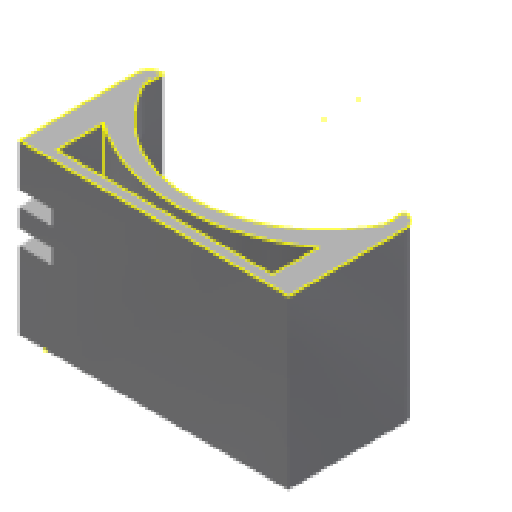
# Autodesk Inventor part: Gehäuse_Kurve
Saved by Autodesk Inventor 2023 (Build 270158000, 158)
## iProperties
Created: 2025-01-24
Part Number: Gehäuse_Kurve
Material: ABS-Kunststoff
Document SubType Name: Modeling
Designer: abdel
Density: 1.06 g/cm^3
Appearance: Glatt - Weiß
Author: abdel
Autodesk Inventor part; units mm, degrees
ref_plane "YZ Plane" through (0, 0, 0) normal (1, 0, 0) x (0, 1, 0)
ref_plane "XY Plane" through (0, 0, 0) normal (0, 0, 1) x (1, 0, 0)
sketch "Skizze1" plane through (0, 0, 0) normal (0, 0, 1) x (1, 0, 0)
  line L0 (20, 16.3) -> (20, 0)
  line L1 (20, 0) -> (-20, 0)
  line L2 (-20, 0) -> (-20, 16.3)
  line L3 (-16, 8.4971) -> (-16, 1.5701)
  line L4 (-16, 1.5701) -> (16, 1.5701)
  line L5 (16, 1.5701) -> (16, 8.4971)
  line L6 (-20, 16.3) -> (-17.85, 16.3)
  line L7 (20, 16.3) -> (17.85, 16.3)
  arc A0 (-16, 8.4971) -> (16, 8.4971) centre (0, 30.4255) ccw
  arc A1 (-17.85, 16.3) -> (17.85, 16.3) centre (0, 25.395) ccw
  line L8 (2.1309, 0) -> (0, 0)
  line L9 (0, 16.2928) -> (2.1309, 16.2928)
  line L10 (2.1309, 16.2928) -> (2.1309, 0)
  line L11 (2.1309, 0) -> (0, 0)
  line L12 (0, 0) -> (0, 16.2928)
  line L13 (37.8691, 16.2928) -> (40, 16.2928)
  line L14 (40, 16.2928) -> (40, 0)
  line L15 (40, 0) -> (37.8691, 0)
  line L16 (37.8691, 0) -> (37.8691, 16.2928)
  line L17 (0, 0) -> (40, 0)
  line L18 (0, 0) -> (0, 12.8953)
  line L19 (40, 0) -> (40, 79)
  arc A2 (2.1309, 16.2928) -> (37.8691, 16.2928) centre (20, 25.8644) ccw
  line L20 (6.1071, 11.1028) -> (5.3563, 11.7632)
  point P0 (0, 8.1464)
  dimension "d27" = 40
  dimension "d28" = 4
  dimension "d58" = 16.3
  dimension "d60" = 126
  dimension "d61" = 2.15
  dimension "d62" = 2.1309
  constraints: 42 end point, 7 point on circle, 6 horizontal, 5 parallel, 4 equal length, 4 point on line, 3 centre point, 3 vertical, 2 midpoint, 2 perpendicular, 1 coincident
  measures "d27" distance of L0.end L1.end
  measures "d28" distance between parallel lines of L0 L5
  measures "d58" distance of L1.end L2.end
  measures "d61" distance of L2.end L6.end
  measures "d62" distance of L9.start L9.end
extrude "Extrusion1" add sketch "Skizze1" along normal blind 25 contours L0 A2 L5 A0 A1 L7 | L0 L1 L10 L4 L5 A2 | A2 A0 L10 A1 | L1 L12 L4 L10 | L10 A0 L12 A1 | L1 L2 L6 A1 L12 A0 L3 L4
sketch "Skizze2" plane through (-20, 16.3, 0) normal (0, 1, 0) x (1, 0, 0)
  line L0 (2.15, 0) -> (0, 0) projected
  line L1 (0, 0) -> (0, -25) projected
  line L2 (2.15, -25) -> (0, -25) projected
  line L3 (2.15, 0) -> (2.15, -25) projected
  point P0 (20, 0)
extrude "Extrusion2" add sketch "Skizze2" along normal blind 3
sketch "Skizze3" plane through (17.85, 16.3, 0) normal (0, 1, 0) x (1, 0, 0)
  line L0 (2.15, 0) -> (0, 0) projected
  line L1 (0, 0) -> (0, -25) projected
  line L2 (2.15, -25) -> (0, -25) projected
  line L3 (2.15, 0) -> (2.15, -25) projected
  point P0 (-17.85, 0)
ref_plane "Arbeitsebene2" through (0, 10, 0) normal (0, 1, 0) x (-1, 0, 0)
extrude "Extrusion3" add sketch "Skizze3" along normal blind 3
sketch "Skizze4" plane through (0, 10, 0) normal (0, 1, 0) x (-1, 0, 0)
  line L0 (-17.85, 0) -> (-17.85, 25) projected
  line L1 (-17.85, 0) -> (17.85, 0) projected
  line L2 (17.85, 0) -> (17.85, 25) projected
  line L3 (-17.85, 25) -> (17.85, 25) projected
  line L4 (-17.85, 0) -> (-17.85, 25) projected
  line L5 (-17.85, 11.4) -> (17.85, 11.4)
  line L6 (-17.85, 13.65) -> (17.85, 13.65)
  line L7 (-17.85, 16.4) -> (17.85, 16.4)
  line L8 (-17.85, 18.65) -> (17.85, 18.65)
  line L9 (-17.85, 25) -> (-20, 25) projected
  point P0 (0, 0)
  point P1 (-17.85, 13.65)
  point P2 (-17.85, 11.4)
  point P3 (-17.85, 18.65)
  point P4 (-17.85, 16.4)
  dimension "d13" = 2.25
  dimension "d14" = 2.25
  dimension "d15" = 25
  dimension "d16" = 2.75
  dimension "d36" = 6.35
  constraints: 8 end point, 8 point on line, 4 horizontal
  measures "d13" distance between parallel lines of L5 L6
  measures "d14" distance between parallel lines of L7 L8
  measures "d15" distance between parallel lines of L1 L3
  measures "d16" distance between parallel lines of L6 L7
  measures "d36" distance between parallel lines of L9 L8
extrude "Extrusion4" cut sketch "Skizze4" along normal mid plane 14 contours L0 L6 L2 L5 | L0 L8 L2 L7
fillet "Rundung2" radius 2 2 edges at (-20, 19.3, 12.5) (20, 19.3, 12.5)
sketch "Skizze5" plane through (-16, 1.5701, 0) normal (1, 0, 0) x (0, 0, -1)
  line L0 (0, 0) -> (0, 6.927) projected
  line L1 (0, 6.927) -> (-25, 6.927) projected
  line L2 (-25, 0) -> (-25, 6.927) projected
  line L3 (0, 0) -> (-25, 0) projected
  point P0 (0, -1.5701)
sketch "Skizze12" plane through (-20, 0, 0) normal (-1, 0, 0) x (0, 0, 1)
  line L0 (0, 0) -> (25, 0) projected
  line L1 (18.65, 6.5) -> (18.65, 12)
  line L2 (13.65, 6.5) -> (13.65, 12)
  line L3 (18.65, 12) -> (16.4, 12)
  line L4 (16.4, 12) -> (16.4, 0)
  line L5 (16.4, 0) -> (18.65, 0)
  line L6 (18.65, 0) -> (18.65, 12)
  line L7 (13.65, 12) -> (11.4, 12)
  line L8 (11.4, 12) -> (11.4, 0)
  line L9 (11.4, 0) -> (13.65, 0)
  line L10 (13.65, 0) -> (13.65, 12)
  point P0 (27, 0)
  point P1 (13.65, 0)
  point P2 (18.65, 0)
  dimension "d52" = 2.75
  dimension "d54" = 2.25
  dimension "d55" = 2.25
  constraints: 20 end point, 4 parallel, 2 horizontal, 2 perpendicular, 2 point on line
  measures "d52" distance between parallel lines of L10 L4
  measures "d54" distance between parallel lines of L8 L10
  measures "d55" distance between parallel lines of L6 L4
extrude "Extrusion10" cut sketch "Skizze12" against normal blind 5
sketch "Skizze13" plane through (0, 0, 25) normal (0, 0, 1) x (1, 0, 0)
  arc A0 (20, 17.3) -> (17.85, 19.3) centre (18, 17.3) ccw projected
  line L0 (17.85, 16.3) -> (17.85, 19.3) projected
  arc A1 (-17.85, 16.3) -> (17.85, 16.3) centre (0, 25.395) ccw projected
  line L1 (-17.85, 16.3) -> (-17.85, 19.3) projected
  arc A2 (-17.85, 19.3) -> (-20, 17.3) centre (-18, 17.3) ccw projected
  line L2 (-20, 0) -> (-20, 17.3) projected
  line L3 (-20, 0) -> (20, 0) projected
  line L4 (20, 0) -> (20, 17.3) projected
  arc A3 (-16, 8.4971) -> (16, 8.4971) centre (0, 30.4255) ccw projected
  line L5 (16, 8.4971) -> (16, 1.5701) projected
  line L6 (16, 1.5701) -> (-16, 1.5701) projected
  line L7 (-16, 1.5701) -> (-16, 8.4971) projected
  point P0 (0, 0)
  constraints: 2 other
